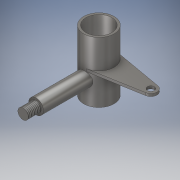
# Autodesk Inventor part: steering_kingpin
Saved by Autodesk Inventor 2019 (Build 230136000, 136)
## iProperties
Created: 2019-04-24
Part Number: steering_kingpin
Material: Steel, Mild
Document SubType Name: Modeling
Designer: callum.snowden
Density: 7.85 g/cm^3
Appearance: Semi-Polished
Author: callum.snowden
Autodesk Inventor part; units mm, degrees
ref_plane "XZ Plane" through (0, 0, 0) normal (0, 1, 0) x (-1, 0, 0)
sketch "Sketch1" plane through (0, 0, 0) normal (0, 1, 0) x (-1, 0, 0)
  line L0 (0, -24.5) -> (0, 24.5) construction
  line L1 (-24.5, 0) -> (24.5, 0) construction
  circle A0 centre (0, 0) radius 17.5
  circle A1 centre (0, 0) radius 15
  dimension "d0" = 35
  dimension "d1" = 30
  constraints: 2 centre point, 2 coincident
  measures "d0" diameter of A0
  measures "d1" diameter of A1
extrude "Extrusion1" add sketch "Sketch1" along normal blind 70
ref_plane "Work Plane4" through (0, 0, 17.5) normal (0, 0, 1) x (1, 0, 0)
sketch "Sketch2" plane through (0, 0, 17.5) normal (0, 0, 1) x (1, 0, 0)
  line L0 (17.5, 70) -> (-17.5, 70) construction
  line L1 (-17.5, 0) -> (17.5, 0) construction
  line L2 (0, 84) -> (0, -14) construction
  circle A0 centre (0, 25) radius 8.5
  point P0 (0, 0)
  dimension "d5" = 17
  dimension "d6" = 25
  constraints: 1 centre point, 1 point on line
  measures "d5" diameter of A0
  measures "d6" distance from line of L1 A0.centre
extrude "Extrusion2" add sketch "Sketch2" along normal blind 55
extrude "Extrusion3" add sketch "Sketch2" against normal up to next
sketch "Sketch3" plane through (0, 25, 72.5) normal (0, 0, 1) x (1, 0, 0)
  circle A0 centre (0, 0) radius 8.5 construction
  circle A1 centre (0, 0) radius 6
  point P0 (0, -25)
  dimension "d11" = 12
  constraints: 1 centre point, 1 coincident
  measures "d11" diameter of A1
extrude "Extrusion4" add sketch "Sketch3" along normal blind 15
thread "Thread1" size "M12x1.75" class "6g" standard "ISO Metric profile" length 15
sketch "Sketch5" plane through (0, 25, 87.5) normal (-1, 0, 0) x (0, 1, 0)
  line L0 (6, 0) -> (6, 15)
  line L1 (6, 15) -> (4.7024, 15)
  line L2 (4.7024, 15) -> (4.7024, 0)
  line L3 (4.7024, 0) -> (6, 0)
  line L4 (0, -23.29) -> (0, 126.3817) projected
  constraints: 8 end point
revolve "Revolution1" [suppressed]
sketch "Sketch6" plane through (0, 25, 87.5) normal (-1, 0, 0) x (0, 1, 0)
  line L0 (6, 0) -> (6, 15)
  line L1 (6, 15) -> (4.7024, 15)
  line L2 (4.7024, 15) -> (4.7024, 0)
  line L3 (4.7024, 0) -> (6, 0)
  line L4 (0, -23.29) -> (0, 126.3817) projected
  constraints: 8 end point
revolve "Revolution2" [suppressed]
sketch "Sketch4" plane through (0, 25, 87.5) normal (1, 0, 0) x (0, 0, -1)
  line L0 (-1.0209, -4.7911) -> (-0.8751, -4.7911) construction
  line L1 (0.1457, -5.9117) -> (-0.0001, -6.1918) construction
  line L2 (-1.7501, -6.1918) -> (-1.8959, -5.9117) construction
  line L3 (-0.7293, -4.7911) -> (-0.8751, -4.511) construction
  line L4 (-0.8751, -4.511) -> (-1.0209, -4.7911) construction
  line L5 (-1.7501, -6.1918) -> (-1.6043, -5.9117) construction
  line L6 (-0.7293, -4.7911) -> (-0.1459, -5.9117)
  line L7 (-1.8959, -5.9117) -> (-1.6043, -5.9117) construction
  arc A0 (-1.8959, -5.9117) -> (-1.7501, -6.0002) centre (-1.7501, -5.8358) ccw construction
  line L8 (0.1457, -5.9117) -> (-0.1459, -5.9117) construction
  line L9 (-1.7501, -6.1918) -> (-1.7501, -5.9117) construction
  line L10 (-0.0001, -6.1918) -> (-0.0001, -5.9117) construction
  line L11 (-0.8751, -4.511) -> (-0.8751, -4.7026) construction
  line L12 (-1.7501, -6.0002) -> (-0.0001, -6.0002)
  arc A1 (-1.7501, -6.0002) -> (-1.6043, -5.9117) centre (-1.7501, -5.8358) ccw
  line L13 (-0.1459, -5.9117) -> (-0.0001, -6.1918) construction
  line L14 (-1.6043, -5.9117) -> (-1.0209, -4.7911)
  line L15 (-0.0001, -0.0002) -> (-0.0001, 0.0177)
  line L16 (-0.0001, 0.0177) -> (-0.0001, -0.0002)
  line L17 (-0.0001, -0.0002) -> (0.0334, -0.0002)
  arc A2 (-0.1459, -5.9117) -> (-0.0001, -6.0002) centre (-0.0001, -5.8358) ccw
  arc A3 (-0.0001, -6.0002) -> (0.1457, -5.9117) centre (-0.0001, -5.8358) ccw construction
  arc A4 (-0.8751, -4.7026) -> (-1.0209, -4.7911) centre (-0.8751, -4.867) ccw
  arc A5 (-0.7293, -4.7911) -> (-0.8751, -4.7026) centre (-0.8751, -4.867) ccw
  line L18 (-0.8751, -4.7026) -> (-0.8751, -4.7911) construction
  line L19 (-0.8751, -4.7911) -> (-0.7293, -4.7911) construction
  dimension "d16" = 55
  dimension "d17" = 0.2802
  dimension "d18" = 0.2802
  dimension "Sketch4_ThreadOffset" = 0
  dimension "Sketch4_MajorRadius" = 6
  dimension "d21" = 1.75
  dimension "Sketch4_MinorRadius" = 4.7024
  constraints: 40 end point, 12 point on circle, 10 parallel, 8 tangent, 6 centre point, 6 collinear, 2 midpoint, 2 point on line, 1 horizontal, 1 perpendicular, 3 other
  measures "d16" angle of L6 L14
  measures "d17" distance of L3.end L0.end
  measures "d18" distance of L1.end L10.end
  measures "Sketch4_ThreadOffset" distance between parallel lines of L15 L10
  measures "Sketch4_MajorRadius" distance from line of L12 L15.start
  measures "d21" distance from line of L1.end L9
  measures "Sketch4_MinorRadius" distance edge to line of A5 L17
coil "Coil1" [suppressed]
ref_plane "Work Plane5" through (17.5, 0, 0) normal (1, 0, 0) x (0, 1, 0)
ref_plane "Work Plane6" through (0, 35, 0) normal (0, -1, 0) x (1, 0, 0)
sketch "Sketch7" plane through (0, 35, 0) normal (0, -1, 0) x (1, 0, 0)
  circle A0 centre (0, 0) radius 15 construction
  line L0 (0, 109.2) -> (0, -38.6167) construction
  line L1 (-24.5, 0) -> (24.5, 0) construction
  arc A1 (61.225, -6.892) -> (61.225, 6.892) centre (60, 0) ccw
  line L2 (3.0625, -17.2299) -> (61.225, -6.892)
  line L3 (3.0625, 17.2299) -> (61.225, 6.892)
  arc A2 (3.0625, -17.2299) -> (3.0625, 17.2299) centre (0, 0) ccw
  circle A3 centre (60, 0) radius 4
  dimension "d35" = 14
  dimension "d36" = 60
  dimension "d37" = 8
  constraints: 4 centre point, 4 end point, 4 point on circle, 4 tangent, 1 coincident, 1 point on line
  measures "d35" diameter of A1
  measures "d36" distance of A1.centre point (0, 0)
  measures "d37" diameter of A3
extrude "Extrusion5" add sketch "Sketch7" along normal mid plane 3
equation "\"d16\" = d23"
equation "\"d17\" = 0.160083 * Sketch4_Pitch"
equation "\"d18\" = 0.160083 * Sketch4_Pitch"
equation "\"d21\" = Sketch4_Pitch"
equation "\"d23\" = 55deg"
equation "\"Sketch4_Pitch\" = 1.75"
body "Solid1"
body "Solid2"
